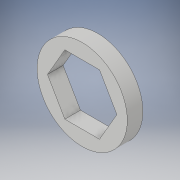
# Autodesk Inventor part: 3D Model Spacer Arm
Saved by Autodesk Inventor 2018 (Build 220112000, 112)
## iProperties
Created: 2019-01-26
Part Number: 3D Model Spacer Arm
Material: Generic
Document SubType Name: Modeling
Designer: Gabriel
Density: 1 g/cm^3
Appearance: Default
Author: Gabriel
Autodesk Inventor part; units mm, degrees
ref_plane "YZ Plane" through (0, 0, 0) normal (1, 0, 0) x (0, 1, 0)
ref_plane "XZ Plane" through (0, 0, 0) normal (0, 1, 0) x (-1, 0, 0)
ref_plane "XY Plane" through (0, 0, 0) normal (0, 0, 1) x (1, 0, 0)
sketch "Sketch1" plane through (0, 0, 0) normal (0, 0, 1) x (1, 0, 0)
  circle A0 centre (0, 0) radius 9.525
  line L0 (0, 0) -> (0, 6.35) construction
  line L1 (3.6695, 6.35) -> (7.334, -0.0028)
  line L2 (7.334, -0.0028) -> (3.6645, -6.3528)
  line L3 (3.6645, -6.3528) -> (-3.6695, -6.35)
  line L4 (-3.6695, -6.35) -> (-7.334, 0.0028)
  line L5 (-7.334, 0.0028) -> (-3.6645, 6.3528)
  line L6 (-3.6645, 6.3528) -> (3.6695, 6.35)
  dimension "d0" = 19.05
  dimension "d1" = 6.35
  constraints: 14 end point, 2 coincident, 1 centre point, 1 vertical, 13 other
  measures "d0" diameter of A0
  measures "d1" distance of L0.start L0.end
extrude "Extrusion1" add sketch "Sketch1" along normal blind 3.302
body "Solid1"
